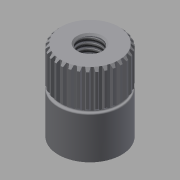
# Autodesk Inventor part: pinion
Saved by Autodesk Inventor 2014 (Build 180170000, 170)
## iProperties
Created: 2013-07-12
Part Number: pinion
Material: Generic
Document SubType Name: Modeling
Designer: Maurice
Density: 1 g/cm^3
Appearance: Default
Author: Maurice
Autodesk Inventor part; units mm, degrees
ref_plane "YZ Plane" through (0, 0, 0) normal (1, 0, 0) x (0, 1, 0)
ref_plane "XZ Plane" through (0, 0, 0) normal (0, 1, 0) x (-1, 0, 0)
ref_plane "XY Plane" through (0, 0, 0) normal (0, 0, 1) x (1, 0, 0)
sketch "Sketch1" plane through (0, 0, 0) normal (0, 1, 0) x (-1, 0, 0)
  arc A0 (0, 2.935) -> (-0.2069, 2.9277) centre (0, 0) ccw
  arc A1 (-0.1, 2.6781) -> (0.1, 2.6781) centre (0, 0) ccw
  line L0 (0.21, 2.935) -> (-0.21, 2.935)
  line L1 (0.1, 2.6781) -> (-0.1, 2.6781)
  line L2 (0.1, 2.6781) -> (0.21, 2.935)
  line L3 (-0.21, 2.935) -> (-0.1, 2.6781)
  arc A2 (0.1, 2.6781) -> (-0.1, 2.6781) centre (0, 0) ccw
  arc A3 (0.2069, 2.9277) -> (0, 2.935) centre (0, 0) ccw
  arc A4 (-0.2069, 2.9277) -> (0.2069, 2.9277) centre (0, 0) ccw
  point P0 (0, 2.6781)
  dimension "d0" = 5.87
  dimension "d1" = 5.36
  dimension "d2" = 0.42
  dimension "d3" = 0.2
  constraints: 10 point on circle, 8 end point, 5 centre point, 3 midpoint, 2 coincident, 2 point on line, 2 vertical alignment, 1 horizontal, 1 parallel
  measures "d0" diameter of A0
  measures "d1" diameter of A1
  measures "d2" distance of L0.start L0.end
  measures "d3" distance of L1.start L1.end
extrude "Extrusion1" add sketch "Sketch1" along normal blind 7.5 contours A3 L2 L1 L3 A0 | L3 A1 L2 A4 | L1 A1
sketch "Sketch2" plane through (0, 7.5, 0) normal (0, 1, 0) x (1, 0, 0)
  line L0 (-0.1, -2.6781) -> (-0.21, -2.935) projected
  line L1 (-0.21, -2.935) -> (0.21, -2.935) projected
  line L2 (0.21, -2.935) -> (0.1, -2.6781) projected
  line L3 (-0.1, -2.6781) -> (0.1, -2.6781) projected
extrude "Extrusion2" cut sketch "Sketch2" against normal blind 3.5
pattern_circular "Circular Pattern1" count 30 over 360 about axis through (0, -10, 0) along (0, 1, 0) of "Extrusion2"
sketch "Sketch3" plane through (0, 0, 0) normal (0, 0, 1) x (1, 0, 0)
  line L0 (2.935, 0) -> (-2.935, 0) construction
  line L1 (-0.4063, 7.5) -> (-0.4063, 4) construction
  line L2 (-0.4063, 4) -> (-0.8111, 4) construction
  line L3 (-0.8111, 4) -> (-0.8111, 7.5) construction
  line L4 (-1.0018, 7.5) -> (-0.8111, 7.5) construction
  line L5 (-1.0018, 7.5) -> (-1.0018, 4) construction
  line L6 (-1.0018, 4) -> (-1.3798, 4) construction
  line L7 (-1.3798, 4) -> (-1.3798, 7.5) construction
  line L8 (-1.5535, 7.5) -> (-1.3798, 7.5) construction
  line L9 (-1.5535, 7.5) -> (-1.5535, 4) construction
  line L10 (-1.5535, 4) -> (-1.8882, 4) construction
  line L11 (-1.8882, 4) -> (-1.8882, 7.5) construction
  line L12 (-2.0373, 7.5) -> (-1.8882, 7.5) construction
  line L13 (-2.0373, 7.5) -> (-2.0373, 4) construction
  line L14 (-2.0373, 4) -> (-2.3141, 4) construction
  line L15 (-2.3141, 4) -> (-2.3141, 7.5) construction
  line L16 (-2.432, 7.5) -> (-2.3141, 7.5) construction
  line L17 (-2.432, 7.5) -> (-2.432, 4) construction
  line L18 (-2.432, 4) -> (-2.6389, 4) construction
  line L19 (-2.6389, 4) -> (-2.6389, 7.5) construction
  line L20 (-2.7205, 7.5) -> (-2.6389, 7.5) construction
  line L21 (-2.7205, 7.5) -> (-2.7205, 4) construction
  line L22 (-2.7205, 4) -> (-2.8483, 4) construction
  line L23 (-2.8483, 4) -> (-2.8483, 7.5) construction
  line L24 (-2.89, 7.5) -> (-2.8483, 7.5) construction
  line L25 (-2.89, 7.5) -> (-2.89, 4) construction
  line L26 (-2.89, 4) -> (-2.9333, 4) construction
  line L27 (-2.9333, 4) -> (-2.9333, 7.5) construction
  line L28 (-2.9333, 7.5) -> (-2.9333, 7.5) construction
  line L29 (-2.9333, 7.5) -> (-2.9333, 4) construction
  line L30 (-2.9333, 4) -> (-2.89, 4) construction
  line L31 (-2.89, 4) -> (-2.89, 7.5) construction
  line L32 (-2.8483, 7.5) -> (-2.89, 7.5) construction
  line L33 (-2.8483, 7.5) -> (-2.8483, 4) construction
  line L34 (-2.8483, 4) -> (-2.7205, 4) construction
  line L35 (-2.7205, 4) -> (-2.7205, 7.5) construction
  line L36 (-2.6389, 7.5) -> (-2.7205, 7.5) construction
  line L37 (-2.6389, 7.5) -> (-2.6389, 4) construction
  line L38 (-2.6389, 4) -> (-2.432, 4) construction
  line L39 (-2.432, 4) -> (-2.432, 7.5) construction
  line L40 (-2.3141, 7.5) -> (-2.432, 7.5) construction
  line L41 (-2.3141, 7.5) -> (-2.3141, 4) construction
  line L42 (-2.3141, 4) -> (-2.0373, 4) construction
  line L43 (-2.0373, 4) -> (-2.0373, 7.5) construction
  line L44 (-1.8882, 7.5) -> (-2.0373, 7.5) construction
  line L45 (-1.8882, 7.5) -> (-1.8882, 4) construction
  line L46 (-1.8882, 4) -> (-1.5535, 4) construction
  line L47 (-1.5535, 4) -> (-1.5535, 7.5) construction
  line L48 (-1.3798, 7.5) -> (-1.5535, 7.5) construction
  line L49 (-1.3798, 7.5) -> (-1.3798, 4) construction
  line L50 (-1.3798, 4) -> (-1.0018, 4) construction
  line L51 (-1.0018, 4) -> (-1.0018, 7.5) construction
  line L52 (-0.8111, 7.5) -> (-1.0018, 7.5) construction
  line L53 (-0.8111, 7.5) -> (-0.8111, 4) construction
  line L54 (-0.8111, 4) -> (-0.4063, 4) construction
  line L55 (-0.4063, 4) -> (-0.4063, 7.5) construction
  line L56 (-0.2069, 7.5) -> (-0.4063, 7.5) construction
  line L57 (-0.2069, 7.5) -> (-0.2069, 4) construction
  line L58 (-0.2069, 4) -> (0.2069, 4) construction
  line L59 (0.2069, 4) -> (0.2069, 7.5) construction
  line L60 (0.4063, 7.5) -> (0.2069, 7.5) construction
  line L61 (0.4063, 7.5) -> (0.4063, 4) construction
  line L62 (0.4063, 4) -> (0.8111, 4) construction
  line L63 (0.8111, 4) -> (0.8111, 7.5) construction
  line L64 (1.0018, 7.5) -> (0.8111, 7.5) construction
  line L65 (1.0018, 7.5) -> (1.0018, 4) construction
  line L66 (1.0018, 4) -> (1.3798, 4) construction
  line L67 (1.3798, 4) -> (1.3798, 7.5) construction
  line L68 (1.5535, 7.5) -> (1.3798, 7.5) construction
  line L69 (1.5535, 7.5) -> (1.5535, 4) construction
  line L70 (1.5535, 4) -> (1.8882, 4) construction
  line L71 (1.8882, 4) -> (1.8882, 7.5) construction
  line L72 (2.0373, 7.5) -> (1.8882, 7.5) construction
  line L73 (2.0373, 7.5) -> (2.0373, 4) construction
  line L74 (2.0373, 4) -> (2.3141, 4) construction
  line L75 (2.3141, 4) -> (2.3141, 7.5) construction
  line L76 (2.432, 7.5) -> (2.3141, 7.5) construction
  line L77 (2.432, 7.5) -> (2.432, 4) construction
  line L78 (2.432, 4) -> (2.6389, 4) construction
  line L79 (2.6389, 4) -> (2.6389, 7.5) construction
  line L80 (2.7205, 7.5) -> (2.6389, 7.5) construction
  line L81 (2.7205, 7.5) -> (2.7205, 4) construction
  line L82 (2.7205, 4) -> (2.8483, 4) construction
  line L83 (2.8483, 4) -> (2.8483, 7.5) construction
  line L84 (2.89, 7.5) -> (2.8483, 7.5) construction
  line L85 (2.89, 7.5) -> (2.89, 4) construction
  line L86 (2.89, 4) -> (2.9333, 4) construction
  line L87 (2.9333, 4) -> (2.9333, 7.5) construction
  line L88 (2.9333, 7.5) -> (2.9333, 7.5) construction
  line L89 (2.9333, 7.5) -> (2.9333, 4) construction
  line L90 (2.9333, 4) -> (2.89, 4) construction
  line L91 (2.89, 4) -> (2.89, 7.5) construction
  line L92 (2.8483, 7.5) -> (2.89, 7.5) construction
  line L93 (2.8483, 7.5) -> (2.8483, 4) construction
  line L94 (2.8483, 4) -> (2.7205, 4) construction
  line L95 (2.7205, 4) -> (2.7205, 7.5) construction
  line L96 (2.6389, 7.5) -> (2.7205, 7.5) construction
  line L97 (2.6389, 7.5) -> (2.6389, 4) construction
  line L98 (2.6389, 4) -> (2.432, 4) construction
  line L99 (2.432, 4) -> (2.432, 7.5) construction
  line L100 (2.3141, 7.5) -> (2.432, 7.5) construction
  line L101 (2.3141, 7.5) -> (2.3141, 4) construction
  line L102 (2.3141, 4) -> (2.0373, 4) construction
  line L103 (2.0373, 4) -> (2.0373, 7.5) construction
  line L104 (1.8882, 7.5) -> (2.0373, 7.5) construction
  line L105 (1.8882, 7.5) -> (1.8882, 4) construction
  line L106 (1.8882, 4) -> (1.5535, 4) construction
  line L107 (1.5535, 4) -> (1.5535, 7.5) construction
  line L108 (1.3798, 7.5) -> (1.5535, 7.5) construction
  line L109 (1.3798, 7.5) -> (1.3798, 4) construction
  line L110 (1.3798, 4) -> (1.0018, 4) construction
  line L111 (1.0018, 4) -> (1.0018, 7.5) construction
  line L112 (0.8111, 7.5) -> (1.0018, 7.5) construction
  line L113 (0.8111, 7.5) -> (0.8111, 4) construction
  line L114 (0.8111, 4) -> (0.4063, 4) construction
  line L115 (0.4063, 4) -> (0.4063, 7.5) construction
  line L116 (0.2069, 7.5) -> (0.4063, 7.5) construction
  line L117 (0.2069, 7.5) -> (0.2069, 4) construction
  line L118 (0.2069, 4) -> (-0.2069, 4) construction
  line L119 (-0.2069, 4) -> (-0.2069, 7.5) construction
  line L120 (-0.4063, 7.5) -> (-0.2069, 7.5) construction
  line L121 (-2.9333, 7.25) -> (-2.6833, 7.5)
  line L122 (-2.9333, 7.25) -> (-2.5797, 7.25) construction
  line L123 (-2.6833, 7.5) -> (-2.4527, 7.7306)
  line L124 (-2.4527, 7.7306) -> (-3.2806, 7.7306)
  line L125 (-2.9333, 7.25) -> (-3.2806, 6.9027)
  line L126 (-3.2806, 6.9027) -> (-3.2806, 7.7306)
  line L127 (-2.9333, 5.75) -> (-3.6243, 5.75) construction
  line L128 (-2.9333, 4.25) -> (-2.6833, 4)
  line L129 (-2.9333, 4.25) -> (-3.2806, 4.5973)
  line L130 (-2.6833, 4) -> (-2.6833, 3.9)
  line L131 (-2.6833, 3.9) -> (-3.2806, 3.9)
  line L132 (-3.2806, 4.5973) -> (-3.2806, 3.9)
  line L133 (0, -1.5461) -> (0, 9.2767) projected
  point P0 (0, 0)
  dimension "d11" = 45
  dimension "d12" = 0.25
  dimension "d13" = 0.1
  constraints: 24 end point, 4 perpendicular, 3 symmetric about line, 2 collinear, 2 point on line, 1 equal length, 1 horizontal, 1 midpoint, 1 parallel
  measures "d11" angle of L122 L121
  measures "d12" distance from line of L29 L121.end
  measures "d13" distance of L128.end L130.end
revolve "Revolution1" cut sketch "Sketch3" angle 360 about axis through (0, -10, 0) along (0, 1, 0)
fillet "Fillet1" radius 0.1 2 edges at (0.2069, 3.9, -2.9277) (2.6833, 3.9, 0)
hole "Hole1" at (0, 7.5, 0) direction (0, -1, 0) diameter 2.113 end through all thread size "M2.6x0.45" class "6H" standard "ISO Metric profile"
chamfer "Chamfer1" distance 0.15 angle 45 1 edges at (0, 7.5, -1.0565)
body "Solid1"
